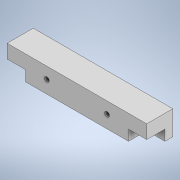
# Autodesk Inventor part: side_bumper_upper
Saved by Autodesk Inventor 2020 (Build 240168000, 168)
## iProperties
Created: 2022-07-20
Part Number: side_bumper_upper
Material: 일반
Document SubType Name: Modeling
Designer: SeungJin
Density: 1 g/cm^3
Appearance: 기본값
Author: SeungJin
Autodesk Inventor part; units mm, degrees
ref_plane "YZ Plane" through (0, 0, 0) normal (1, 0, 0) x (0, 1, 0)
ref_plane "XZ Plane" through (0, 0, 0) normal (0, 1, 0) x (-1, 0, 0)
ref_plane "XY Plane" through (0, 0, 0) normal (0, 0, 1) x (1, 0, 0)
ref_plane "작업 평면1" through (-180.5399, 22.5444, -43) normal (0, 0, 1) x (1, 0, 0)
sketch "스케치3" plane through (-180.5399, 22.5444, -43) normal (0, 0, 1) x (1, 0, 0)
  line L0 (-30.73, 0) -> (-30.73, -60)
  line L1 (199.27, 0) -> (199.27, -60)
  line L2 (-30.73, 0) -> (199.27, 0)
  line L3 (-30.73, -60) -> (199.27, -60)
  line L4 (-0.73, 0) -> (-0.73, -60)
  line L5 (169.27, 0) -> (169.27, -60)
  line L6 (199.27, -40) -> (-30.73, -40)
  dimension "d37" = 230
  dimension "d38" = 60
  dimension "d40" = 30
  dimension "d41" = 30
  dimension "d50" = 20
  constraints: 14 end point, 6 point on line, 3 perpendicular, 2 horizontal, 2 vertical, 1 other
  measures "d37" distance of L0.start L1.start
  measures "d38" distance of L0.start L0.end
  measures "d40" distance between parallel lines of L0 L4
  measures "d41" distance between parallel lines of L5 L1
  measures "d50" distance between parallel lines of L3 L6
extrude "돌출3" add sketch "스케치3" along normal blind 13 contours L2 L4 L6 L0 | L2 L5 L6 L4 | L2 L1 L6 L5
ref_plane "작업 평면2" through (-180.5399, 22.5444, -30) normal (0, 0, 1) x (1, 0, 0)
sketch "스케치4" plane through (-180.5399, 22.5444, -30) normal (0, 0, 1) x (1, 0, 0)
  line L0 (-0.73, -22.544) -> (-30.73, -22.544)
  line L1 (-30.73, 0) -> (-30.73, -40) projected
  line L2 (199.27, -40) -> (199.27, 0) projected
  line L3 (199.27, 0) -> (-30.73, 0) projected
  line L4 (-0.73, -40) -> (-0.73, 0)
  line L5 (169.27, -40) -> (169.27, 0)
  line L6 (169.27, -22.544) -> (199.27, -22.544)
  line L7 (199.27, -60) -> (199.27, 0) projected
  line L8 (-30.73, -40) -> (199.27, -40) projected
  point P0 (-0.73, -40)
  point P1 (169.27, -40)
  dimension "d42" = 22.544
  dimension "d43" = 30
  dimension "d44" = 30
  dimension "d45" = 22.544
  constraints: 8 end point, 8 point on line, 3 perpendicular
  measures "d42" distance between parallel lines of L3 L0
  measures "d43" distance between parallel lines of L1 L4
  measures "d44" distance between parallel lines of L2 L5
  measures "d45" distance between parallel lines of L3 L6
extrude "돌출4" add sketch "스케치4" along normal blind 30 contours L4 L3 L5 L8 | L0 L1 L3 L4 | L3 L2 L6 L5
sketch "스케치5" plane through (-180.5399, 22.5444, 0) normal (0, 0, 1) x (1, 0, 0)
  line L0 (-30.73, -22.544) -> (-0.73, -22.544) projected
  line L1 (199.27, -22.544) -> (199.27, 0) projected
  line L2 (199.27, 0) -> (-30.73, 0) projected
  line L3 (-30.73, 0) -> (-30.73, -22.544) projected
  line L4 (-0.73, -22.544) -> (-0.73, -40) projected
  line L5 (169.27, -40) -> (169.27, -22.544) projected
  line L6 (169.27, -22.544) -> (199.27, -22.544) projected
  line L7 (-0.73, -40) -> (169.27, -40) projected
  point P0 (180.5399, -22.5444)
  point P1 (34.635, -19)
  point P2 (133.9049, -19)
  dimension "d46" = 19
  dimension "d47" = 19
  dimension "d48" = 35.365
  dimension "d49" = 35.365
  measures "d46" distance from line of L2 point (133.905, -19)
  measures "d47" distance from line of L2 point (34.635, -19)
  measures "d48" distance from line of L5 point (133.905, -19)
  measures "d49" distance from line of point (34.635, -19) L4
hole "구멍1" at (-145.9049, 3.5444, 0) at (-46.635, 3.5444, 0) direction (0, 0, -1) diameter 4.5 end through all counterbore diameter 8 counterbore depth 25 clearance for "Hex Head Cap Screw ISO 24017" size "M4" standard "ISO"
ref_plane "작업 평면4" through (-180.5399, 22.5444, -43) normal (0, 0, -1) x (-1, 0, 0)
sketch "스케치6" plane through (-180.5399, 22.5444, -43) normal (0, 0, -1) x (-1, 0, 0)
  circle A0 centre (-34.635, -19) radius 2.25 projected
  circle A1 centre (-133.9049, -19) radius 2.25 projected
  line L0 (30.73, 0) -> (30.73, -40) projected
  line L1 (-199.27, 0) -> (30.73, 0) projected
  line L2 (-199.27, -40) -> (-199.27, 0) projected
  line L3 (30.73, -40) -> (-199.27, -40) projected
  line L4 (-169.27, -22.544) -> (-169.27, -40) projected
  line L5 (-199.27, -22.544) -> (-169.27, -22.544) projected
  line L6 (0.73, -22.544) -> (30.73, -22.544) projected
  line L7 (0.73, -40) -> (0.73, -22.544) projected
  point P0 (-184.27, -32.544)
  point P1 (15.73, -32.544)
  point P2 (15.73, -22.544)
  point P3 (-184.27, -22.544)
  dimension "d51" = 10
  dimension "d52" = 10
  constraints: 2 midpoint, 2 vertical alignment
  measures "d51" distance from line of L5 point (-184.27, -32.544)
  measures "d52" distance from line of L6 point (15.73, -32.544)
hole "구멍2" at (3.73, -9.9996, -43) at (-196.27, -9.9996, -43) direction (0, 0, 1) diameter 4.5 end through all counterbore diameter 8 counterbore depth 5 clearance for "Hex Head Cap Screw ISO 24017" size "M4" standard "ISO"
